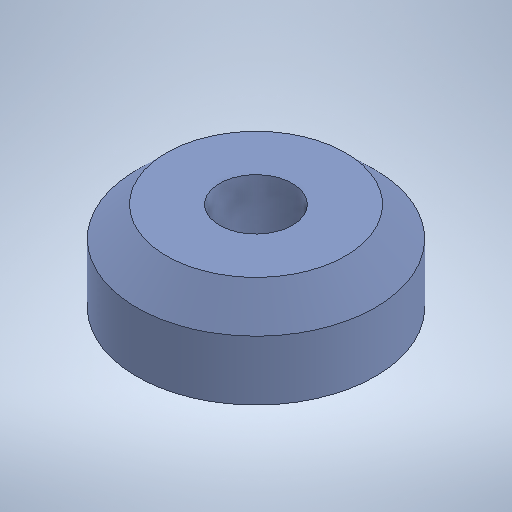
# Autodesk Inventor part: peça_001_001
Saved by Autodesk Inventor 2026 (Build 300175000, 175)
## iProperties
Created: 2025-04-08
Part Number: peça_001_001
Material: Rubber
Document SubType Name: Modeling
Designer: Carlos Dias
Density: 0.93 g/cm^3
Appearance: Rubber - Blue
Author: Carlos Dias
Autodesk Inventor part; units mm, degrees
sketch "Sketch1" plane through (0, 0, 0) normal (0, 0, 1) x (1, 0, 0)
  line L0 (-15, 15) -> (-20, 10)
  line L1 (-20, 10) -> (-20, 0)
  line L2 (-15, 15) -> (0, 15)
  line L3 (0, 15) -> (0, 0)
  line L4 (-20, 0) -> (0, 0)
  dimension "d0" = 20
  dimension "d1" = 10
  dimension "d2" = 135
  dimension "d3" = 5
  constraints: 10 end point, 2 horizontal, 2 vertical, 1 coincident, 1 horizontal alignment, 1 vertical alignment
  measures "d0" distance of point (0, 0) L1.end
  measures "d1" distance of L0.end L1.end
  measures "d2" angle of L1 L0
  measures "d3" horizontal distance of L0.start L0.end
revolve "Revolution1" add sketch "Sketch1" angle 360 mid plane about axis through (0, 15, 0) along (0, -1, 0)
sketch "Sketch2" plane through (0, 15, 0) normal (0, 1, 0) x (1, 0, 0)
  circle A0 centre (0, 0) radius 6.1
  dimension "d5" = 12.2
  constraints: 1 centre point, 1 coincident
  measures "d5" diameter of A0
extrude "Extrusion1" cut sketch "Sketch2" against normal through all
sketch "Sketch3" plane through (0, 0, 0) normal (0, -1, 0) x (1, 0, 0)
  line L0 (0, 10.2) -> (8.8335, 5.1)
  line L1 (8.8335, 5.1) -> (8.8335, -5.1)
  line L2 (8.8335, -5.1) -> (0, -10.2)
  line L3 (0, -10.2) -> (-8.8335, -5.1)
  line L4 (-8.8335, -5.1) -> (-8.8335, 5.1)
  line L5 (-8.8335, 5.1) -> (0, 10.2)
  point P0 (0, 0)
  point P1 (0, 0)
  dimension "d8" = 10.2
  constraints: 12 end point, 1 coincident, 1 vertical, 13 other
  measures "d8" distance of L3.end L4.end
extrude "Extrusion2" cut sketch "Sketch3" against normal blind 5
body "Solid1"
